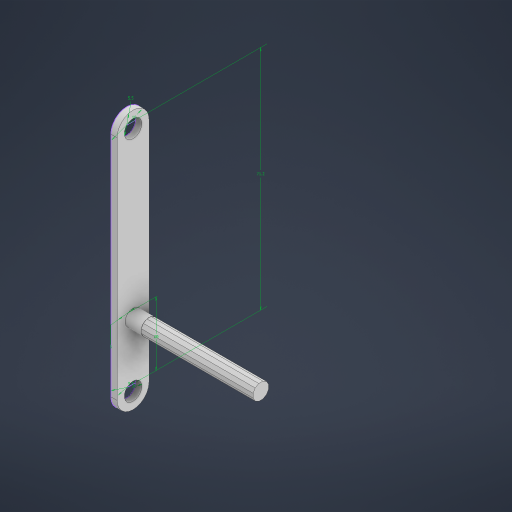
# Autodesk Inventor part: gunholder_v3 R
Saved by Autodesk Inventor 2024.1 (Build 281209000, 209)
## iProperties
Created: 2023-07-11
Part Number: gunholder_v3 R
Material: 일반
Document SubType Name: Modeling
Designer: 6gioc
Density: 1 g/cm^3
Appearance: 기본값
Author: 6gioc
## iProperties of the stored document gunholder_v3 R_3D 인쇄.ipt
Created: 2023-09-27
Part Number: gunholder_v3 R_3D 인쇄
Material: 일반
Document SubType Name: Modeling
Designer: 6gioc
Density: 1 g/cm^3
Appearance: 기본값
Author: 6gioc
Autodesk Inventor part; units mm, degrees
ref_plane "YZ Plane" through (0, 0, 0) normal (1, 0, 0) x (0, 1, 0)
ref_plane "XZ Plane" through (0, 0, 0) normal (0, 1, 0) x (-1, 0, 0)
ref_plane "XY Plane" through (0, 0, 0) normal (0, 0, 1) x (1, 0, 0)
sketch "스케치1" plane through (0, 0, 0) normal (1, 0, 0) x (0, 1, 0)
  line L0 (2.4148, 0.647) -> (2.4148, -0.647)
  line L1 (1.7678, 1.7678) -> (2.4148, 0.647)
  line L2 (2.4148, -0.647) -> (1.7678, -1.7678)
  line L3 (1.7678, -1.7678) -> (0.647, -2.4148)
  line L4 (-0.647, 2.4148) -> (0.647, 2.4148)
  line L5 (0.647, -2.4148) -> (-0.647, -2.4148)
  circle A0 centre (0, 0) radius 2.5
  line L6 (0.647, 2.4148) -> (1.7678, 1.7678)
  line L7 (-0.647, -2.4148) -> (-1.7678, -1.7678)
  line L8 (-1.7678, -1.7678) -> (-2.4148, -0.647)
  line L9 (-2.4148, -0.647) -> (-2.4148, 0.647)
  line L10 (-2.4148, 0.647) -> (-1.7678, 1.7678)
  line L11 (-1.7678, 1.7678) -> (-0.647, 2.4148)
  circle A1 centre (-20, 0) radius 2.75
  circle A2 centre (-20, 0) radius 5
  circle A3 centre (51.2, 0) radius 5
  circle A4 centre (51.2, 0) radius 2.75
  line L12 (51.2, 5) -> (-20, 5)
  line L13 (-20, 5) -> (-20, -5)
  line L14 (-20, -5) -> (51.2, -5)
  line L15 (51.2, -5) -> (51.2, 5)
  point P0 (2.5, 0)
  dimension "d0" = 5
  dimension "d2" = 10
  dimension "d4" = 10
  dimension "d1" = 5.5
  dimension "d3" = 20
  dimension "d5" = 71.2
  dimension "d6" = 5.5
  constraints: 32 end point, 7 coincident, 2 centre point, 2 parallel, 1 horizontal, 1 perpendicular, 35 other
  measures "d1" diameter of A1
  measures "d3" distance of point (0, 0) A1.centre
  measures "d5" distance of point (-20, 0) point (51.2, 0)
  measures "d6" diameter of A4
extrude "돌출1" add sketch "스케치1" along normal blind 2 contours A1 L13 A2 | A1 L13 A2 | L12 A3 L14 A2 | L15 A4 A3 | A3 L15 A4
extrude "돌출2" add sketch "스케치1" along normal blind 7 contours A0 L0 | L1 A0 | A0 L2 | L6 A0 | A0 L3 | L4 A0 | A0 L5 | L11 A0 | A0 L7 | L10 A0 | A0 L8 | L9 A0
extrude "돌출3" add sketch "스케치1" along normal blind 42 contours L0 L2 L3 L5 L7 L8 L9 L10 L11 L4 L6 L1
